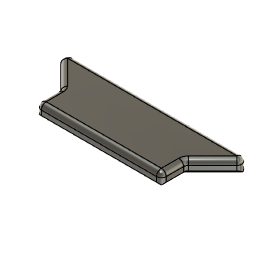
connect test (Autodesk Fusion 360 design; units mm, degrees)
Autodesk Fusion 360 part; units mm, degrees
sketch "Sketch1" plane through (0, 0, 0) normal (0, 0, 1) x (1, 0, 0)
  line L0 (0, 0) -> (-26, 0)
  line L1 (0, 0) -> (26, 0)
  line L2 (0, 0) -> (0, 15) construction
  line L3 (0, 15) -> (41, 15)
  line L4 (0, 15) -> (-41, 15)
  line L5 (-41, 15) -> (-26, 0)
  line L6 (26, 0) -> (41, 15)
  line L7 (25.7929, 0.5) -> (39.7929, 14.5)
  line L8 (0, 14.5) -> (39.7929, 14.5)
  line L9 (0, 14.5) -> (-39.7929, 14.5)
  line L10 (-39.7929, 14.5) -> (-25.7929, 0.5)
  line L11 (0, 0.5) -> (-25.7929, 0.5)
  line L12 (0, 0.5) -> (25.7929, 0.5)
  dimension "d1" = 26
  dimension "d2" = 26
  dimension "d3" = 15
  dimension "d4" = 41
  dimension "d5" = 41
  dimension "d6" = 0.5
  constraint coincident L0.start L1.start
  constraint horizontal L0
  constraint parallel L0 L1
  constraint perpendicular L0 L2
  constraint perpendicular L2 L3
  constraint perpendicular L2 L4
  measures "d1" distance of L0.start L0.end
  measures "d2" distance of L0.start L1.end
  measures "d3" distance of L0.start L2.end
  measures "d4" distance of L2.end L3.end
  measures "d5" distance of L2.end L4.end
extrude "Extrude1" add sketch "Sketch1" along normal blind 5 contours L7 L8 L9 L10 L11 L12
extrude "Extrude2" add 2 faces at (8.5976, 0.5, 1.6667) (-8.5976, 0.5, 1.6667) along direction (0, -1, 0) blind 10
chamfer "Chamfer1" distance 1 angle 45 6 edges at (25.7929, -4.5, 0) (32.7929, 7.5, 0) (0, -9.5, 0) (-25.7929, -4.5, 0) (-32.7929, 7.5, 0) (0, 14.5, 0)
fillet "Fillet1" radius 2 6 edges at (39.7929, 14.5, 3) (25.7929, 0.5, 3) (25.7929, -9.5, 3) (-39.7929, 14.5, 3) (-25.7929, 0.5, 3) (-25.7929, -9.5, 3) 1 faces at (-8.5976, 9.8333, 5)
equation "d1 = ( 52 / 2 ) * 1 mm"
equation "d2 = d1"
equation "d4 = d1 + 15 mm"
equation "d5 = d4"
